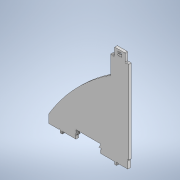
# Autodesk Inventor part: Support D - V2
Saved by Autodesk Inventor 2020 (Build 240168000, 168)
## iProperties
Created: 2020-07-22
Part Number: Support D - V2
Material: Generic
Document SubType Name: Modeling
Designer: Dan Wikman
Density: 1 g/cm^3
Appearance: Default
Author: Dan Wikman
Autodesk Inventor part; units mm, degrees
ref_plane "YZ Plane" through (0, 0, 0) normal (1, 0, 0) x (0, 1, 0)
ref_plane "XZ Plane" through (0, 0, 0) normal (0, 1, 0) x (-1, 0, 0)
ref_plane "XY Plane" through (0, 0, 0) normal (0, 0, 1) x (1, 0, 0)
sketch "Sketch1" plane through (0, 0, 0) normal (0, 0, 1) x (1, 0, 0)
  line L0 (-150, -512.3475) -> (-150, -323.3356) construction
  line L1 (-472.3938, -281.6809) -> (-252.3938, -281.6809) construction
  line L2 (-489.0365, 251.6809) -> (-252.3938, 251.6809) construction
  line L3 (-472.3938, 281.6809) -> (-252.3938, 281.6809) construction
  line L4 (-472.3938, -251.6809) -> (-252.3938, -251.6809) construction
  line L5 (-356.435, 15) -> (-576.435, 15) construction
  line L6 (-472.3938, -281.6809) -> (-472.3938, -251.6809) construction
  line L7 (-252.3938, -281.6809) -> (-252.3938, -251.6809) construction
  line L8 (-252.3938, 278.1809) -> (-252.3938, 251.6809) construction
  line L9 (-472.3938, 281.6809) -> (-472.3938, 251.6809) construction
  line L10 (-356.435, 15) -> (-356.435, -15) construction
  line L11 (-356.435, -15) -> (-576.435, -15) construction
  line L12 (-576.435, -15) -> (-576.435, 15) construction
  arc A0 (-150, -323.3356) -> (0, -356.435) centre (0, 0) ccw construction
  arc A1 (-156.5, -512.3475) -> (-160, -512.3475) centre (-158.25, -512.3475) ccw construction
  arc A2 (-190, -512.3475) -> (-193.5, -512.3475) centre (-191.75, -512.3475) ccw construction
  line L13 (-178.75, -519.0975) -> (-175, -519.0975) construction
  line L14 (-178.75, -529.0975) -> (-175, -529.0975) construction
  line L15 (-175, -519.0975) -> (-175, -529.0975) construction
  arc A3 (-178.75, -519.0975) -> (-178.75, -522.5975) centre (-178.75, -520.8475) ccw construction
  arc A4 (-178.75, -525.5975) -> (-178.75, -529.0975) centre (-178.75, -527.3475) ccw construction
  line L16 (-171.25, -519.0975) -> (-175, -519.0975) construction
  line L17 (-171.25, -529.0975) -> (-175, -529.0975) construction
  arc A5 (-171.25, -522.5975) -> (-171.25, -519.0975) centre (-171.25, -520.8475) ccw construction
  arc A6 (-171.25, -529.0975) -> (-171.25, -525.5975) centre (-171.25, -527.3475) ccw construction
  line L18 (-252.3938, 251.6809) -> (-489.0365, 251.6809) construction
  arc A7 (-334.9122, -265.623) -> (-335.582, -268.123) centre (-330.582, -268.123) ccw construction
  line L19 (-328.3782, -254.3059) -> (-334.9122, -265.623) construction
  arc A8 (-328.3782, -254.3059) -> (-329.8938, -251.6809) centre (-329.8938, -253.4309) ccw construction
  line L20 (-329.8938, -251.6809) -> (-394.8938, -251.6809) construction
  line L21 (-362.3938, -251.6809) -> (-362.3938, -293.6041) construction
  arc A9 (-389.2055, -268.123) -> (-389.8754, -265.623) centre (-394.2055, -268.123) ccw construction
  arc A10 (-394.8938, -251.6809) -> (-396.4093, -254.3059) centre (-394.8938, -253.4309) ccw construction
  line L22 (-396.4093, -254.3059) -> (-389.8754, -265.623) construction
  arc A11 (-389.2055, -291.6809) -> (-389.2055, -288.1809) centre (-389.2055, -289.9309) ccw construction
  line L23 (-389.2055, -291.6809) -> (-396.7055, -291.6809) construction
  line L24 (-396.7055, -281.6809) -> (-472.3938, -281.6809) construction
  line L25 (-328.082, -281.6809) -> (-252.3938, -281.6809) construction
  line L26 (-252.3938, -287.3475) -> (-210.8964, -287.3475) construction
  arc A12 (-210.8964, -287.3475) -> (-150, -323.3356) centre (0, 0) ccw construction
  arc A13 (-472.3938, -281.6809) -> (-246.475, -491.6809) centre (0, 0) ccw construction
  line L27 (-171.25, -436.0915) -> (-171.25, -399.5915) construction
  line L28 (-178.75, -436.0915) -> (-178.75, -399.5915) construction
  line L29 (-177, -437.8415) -> (-173, -437.8415) construction
  line L30 (-177, -397.8415) -> (-173, -397.8415) construction
  arc A14 (-177, -397.8415) -> (-178.75, -399.5915) centre (-177, -399.5915) ccw construction
  arc A15 (-178.75, -436.0915) -> (-177, -437.8415) centre (-177, -436.0915) ccw construction
  arc A16 (-173, -437.8415) -> (-171.25, -436.0915) centre (-173, -436.0915) ccw construction
  arc A17 (-171.25, -399.5915) -> (-173, -397.8415) centre (-173, -399.5915) ccw construction
  line L31 (-200, -512.3475) -> (-200, -491.6809) construction
  arc A18 (-200, -491.6809) -> (-203.5, -491.6809) centre (-201.75, -491.6809) ccw construction
  line L32 (-160, -512.3475) -> (-160, -532.5975) construction
  line L33 (-161.75, -534.3475) -> (-188.25, -534.3475) construction
  line L34 (-190, -532.5975) -> (-190, -512.3475) construction
  line L35 (-171.25, -522.5975) -> (-171.25, -525.5975) construction
  line L36 (-178.75, -522.5975) -> (-178.75, -525.5975) construction
  arc A19 (-190, -532.5975) -> (-188.25, -534.3475) centre (-188.25, -532.5975) ccw construction
  arc A20 (-161.75, -534.3475) -> (-160, -532.5975) centre (-161.75, -532.5975) ccw construction
  line L37 (-156.5, -512.3475) -> (-150, -512.3475) construction
  line L38 (-193.5, -512.3475) -> (-200, -512.3475) construction
  line L39 (-203.5, -491.6809) -> (-246.475, -491.6809) construction
  arc A21 (-396.7055, -288.1809) -> (-396.7055, -291.6809) centre (-396.7055, -289.9309) ccw construction
  line L40 (-396.7055, -281.6809) -> (-396.7055, -288.1809) construction
  line L41 (-389.2055, -288.1809) -> (-389.2055, -268.123) construction
  arc A22 (-335.582, -288.1809) -> (-335.582, -291.6809) centre (-335.582, -289.9309) ccw construction
  line L42 (-335.582, -291.6809) -> (-328.082, -291.6809) construction
  arc A23 (-328.082, -291.6809) -> (-328.082, -288.1809) centre (-328.082, -289.9309) ccw construction
  line L43 (-328.082, -281.6809) -> (-328.082, -288.1809) construction
  line L44 (-335.582, -288.1809) -> (-335.582, -268.123) construction
  arc A24 (-252.3938, -283.8475) -> (-252.3938, -287.3475) centre (-252.3938, -285.5975) ccw construction
  line L45 (-252.3938, -283.8475) -> (-252.3938, -281.6809) construction
  arc A25 (-479.7691, -25) -> (-479.7691, -21.5) centre (-479.7691, -23.25) ccw construction
  arc A26 (-479.7691, -1.4421) -> (-480.4389, 1.0579) centre (-484.7691, -1.4421) ccw construction
  line L46 (-486.9729, 12.375) -> (-480.4389, 1.0579) construction
  arc A27 (-485.4573, 15) -> (-486.9729, 12.375) centre (-485.4573, 13.25) ccw construction
  line L47 (-420.4573, 15) -> (-485.4573, 15) construction
  arc A28 (-425.4757, 1.0579) -> (-426.1456, -1.4421) centre (-421.1456, -1.4421) ccw construction
  arc A29 (-418.9418, 12.375) -> (-420.4573, 15) centre (-420.4573, 13.25) ccw construction
  line L48 (-418.9418, 12.375) -> (-425.4757, 1.0579) construction
  line L49 (-452.9573, 15) -> (-452.9573, -26.9232) construction
  line L50 (-479.7691, -25) -> (-487.2691, -25) construction
  line L51 (-487.2691, -15) -> (-549.7954, -15) construction
  arc A30 (-487.2691, -21.5) -> (-487.2691, -25) centre (-487.2691, -23.25) ccw construction
  line L52 (-487.2691, -15) -> (-487.2691, -21.5) construction
  line L53 (-479.7691, -21.5) -> (-479.7691, -1.4421) construction
  line L54 (-426.1456, -21.5) -> (-426.1456, -1.4421) construction
  arc A31 (-426.1456, -21.5) -> (-426.1456, -25) centre (-426.1456, -23.25) ccw construction
  line L55 (-426.1456, -25) -> (-418.6456, -25) construction
  arc A32 (-418.6456, -25) -> (-418.6456, -21.5) centre (-418.6456, -23.25) ccw construction
  line L56 (-418.6456, -15) -> (-418.6456, -21.5) construction
  line L57 (276.2049, -135.3556) -> (280.6774, -127.609)
  line L58 (279.2083, -124.984) -> (246.5502, -124.984)
  arc A33 (319.0505, -151.484) -> (319.0505, -147.984) centre (319.0505, -149.734) ccw
  arc A34 (328.5505, -147.9841) -> (325.0505, -147.9841) centre (326.8005, -147.9841) ccw
  line L59 (319.0505, -147.984) -> (280.8619, -147.984)
  arc A35 (214.0502, -164.7817) -> (212.5346, -167.4067) centre (214.0502, -166.5317) ccw
  arc A36 (280.5657, -167.4067) -> (279.0502, -164.7817) centre (279.0502, -166.5317) ccw
  arc A37 (274.0318, -178.7238) -> (273.3619, -181.2238) centre (278.3619, -181.2238) ccw
  line L60 (280.5657, -167.4067) -> (274.0318, -178.7238)
  line L61 (273.3619, -201.2817) -> (273.3619, -181.2238)
  arc A38 (273.3619, -201.2817) -> (273.3619, -204.7817) centre (273.3619, -203.0317) ccw
  line L62 (273.3619, -204.7817) -> (280.8619, -204.7817)
  arc A39 (280.8619, -204.7817) -> (280.8619, -201.2817) centre (280.8619, -203.0317) ccw
  line L63 (280.8619, -194.7817) -> (280.8619, -201.2817)
  line L64 (212.2384, -194.7817) -> (212.2384, -201.2817)
  arc A40 (212.2384, -201.2817) -> (212.2384, -204.7817) centre (212.2384, -203.0317) ccw
  arc A41 (219.7384, -204.7817) -> (219.7384, -201.2817) centre (219.7384, -203.0317) ccw
  line L65 (279.0502, -164.7817) -> (214.0502, -164.7817)
  line L66 (219.7384, -201.2817) -> (219.7384, -181.2238)
  line L67 (219.7384, -204.7817) -> (212.2384, -204.7817)
  arc A42 (219.7384, -181.2238) -> (219.0686, -178.7238) centre (214.7384, -181.2238) ccw
  line L68 (212.5346, -167.4067) -> (219.0686, -178.7238)
  line L69 (212.2384, -194.7817) -> (136.5502, -194.7817)
  line L70 (280.8619, -194.7817) -> (356.5502, -194.7817)
  line L71 (325.0505, -147.9841) -> (325.0505, -154.9841)
  line L72 (325.0505, -154.9841) -> (319.0505, -154.9841)
  line L73 (319.0505, -151.484) -> (319.0505, -154.9841)
  line L74 (246.5502, -124.984) -> (246.5502, -110.6064)
  arc A43 (280.6774, -127.609) -> (279.2083, -124.984) centre (279.1622, -126.7334) ccw
  arc A44 (280.8619, -138.8556) -> (280.8619, -135.3556) centre (280.8619, -137.1056) ccw
  line L75 (276.2049, -135.3556) -> (280.8619, -135.3556)
  line L76 (246.5502, -164.7817) -> (246.5502, -170.2759)
  line L77 (280.8619, -147.984) -> (280.8619, -138.8556)
  arc A45 (168.0499, -147.9841) -> (164.5499, -147.9841) centre (166.2999, -147.9841) ccw
  arc A46 (174.0499, -147.984) -> (174.0499, -151.484) centre (174.0499, -149.734) ccw
  line L78 (213.8921, -124.984) -> (246.5502, -124.984)
  line L79 (174.0499, -147.984) -> (212.2384, -147.984)
  line L80 (216.8955, -135.3556) -> (212.423, -127.609)
  line L81 (168.0499, -147.9841) -> (168.0499, -154.9841)
  line L82 (168.0499, -154.9841) -> (174.0499, -154.9841)
  line L83 (174.0499, -151.484) -> (174.0499, -154.9841)
  arc A47 (213.8921, -124.984) -> (212.423, -127.609) centre (213.9382, -126.7334) ccw
  arc A48 (212.2384, -135.3556) -> (212.2384, -138.8556) centre (212.2384, -137.1056) ccw
  line L84 (216.8955, -135.3556) -> (212.2384, -135.3556)
  line L85 (212.2384, -147.984) -> (212.2384, -138.8556)
  arc A49 (-280.3963, -274.7808) -> (-283.8935, -274.681) centre (-282.1435, -274.681) ccw construction
  arc A50 (-289.8935, -278.1809) -> (-289.8935, -274.6809) centre (-289.8935, -276.4309) ccw construction
  line L86 (-329.7357, -251.6809) -> (-362.3938, -251.6809) construction
  line L87 (-289.8935, -274.6809) -> (-328.082, -274.6809) construction
  line L88 (-332.7391, -262.0525) -> (-328.2666, -254.3059) construction
  line L89 (-283.8935, -274.681) -> (-283.8935, -281.681) construction
  line L90 (-283.8935, -281.681) -> (-289.8935, -281.681) construction
  line L91 (-289.8935, -278.1809) -> (-289.8935, -281.681) construction
  arc A51 (-328.2666, -254.3059) -> (-329.7357, -251.6809) centre (-329.7818, -253.4303) ccw construction
  arc A52 (-328.082, -265.5525) -> (-328.082, -262.0525) centre (-328.082, -263.8025) ccw construction
  line L92 (-332.7391, -262.0525) -> (-328.082, -262.0525) construction
  line L93 (-328.082, -274.6809) -> (-328.082, -265.5525) construction
  line L94 (-392.0485, -262.0525) -> (-396.7055, -262.0525) construction
  arc A53 (-396.7055, -262.0525) -> (-396.7055, -265.5525) centre (-396.7055, -263.8025) ccw construction
  line L95 (-392.0485, -262.0525) -> (-396.521, -254.3059) construction
  arc A54 (-395.0519, -251.6809) -> (-396.521, -254.3059) centre (-395.0058, -253.4303) ccw construction
  line L96 (-396.7055, -274.6809) -> (-396.7055, -265.5525) construction
  line L97 (-434.8941, -278.1809) -> (-434.8941, -281.681) construction
  line L98 (-434.8941, -274.6809) -> (-396.7055, -274.6809) construction
  arc A55 (-434.8941, -274.6809) -> (-434.8941, -278.1809) centre (-434.8941, -276.4309) ccw construction
  line L99 (-440.8941, -281.681) -> (-434.8941, -281.681) construction
  line L100 (-440.8941, -274.681) -> (-440.8941, -281.681) construction
  arc A56 (-440.8941, -274.681) -> (-444.3912, -274.7808) centre (-442.6441, -274.681) ccw construction
  line L101 (-395.0519, -251.6809) -> (-362.3938, -251.6809) construction
  line L102 (-444.3912, -274.7808) -> (-476.4404, -274.7808) construction
  arc A57 (-355.7859, -21.5) -> (-227.0273, -274.7808) centre (0, 0) ccw construction
  arc A58 (-549.7954, -15) -> (-476.4404, -274.7808) centre (0, 0) ccw construction
  line L103 (-280.3963, -274.7808) -> (-227.0273, -274.7808) construction
  line L104 (-364.1192, -15) -> (-364.1192, -18) construction
  arc A59 (-364.1192, -18) -> (-364.1192, -21.5) centre (-364.1192, -19.75) ccw construction
  line L105 (-364.1192, -21.5) -> (-355.7859, -21.5) construction
  line L106 (-356.1192, -15) -> (-356.435, -15) construction
  line L107 (-364.1192, -15) -> (-549.7954, -15) construction
  line L108 (-418.6456, -15) -> (-364.1192, -15) construction
  arc A60 (-370.957, -8.0002) -> (-374.457, -8.0002) centre (-372.707, -8.0002) ccw construction
  arc A61 (-380.457, -11.5) -> (-380.457, -8) centre (-380.457, -9.75) ccw construction
  line L109 (-420.2992, 15) -> (-452.9573, 15) construction
  line L110 (-380.457, -8) -> (-418.6456, -8) construction
  line L111 (-423.3026, 4.6284) -> (-418.8301, 12.375) construction
  line L112 (-374.457, -8.0002) -> (-374.457, -15.0002) construction
  line L113 (-374.457, -15.0002) -> (-380.457, -15.0002) construction
  line L114 (-380.457, -11.5) -> (-380.457, -15.0002) construction
  line L115 (-452.9573, 15) -> (-452.9573, 29.3776) construction
  arc A62 (-418.8301, 12.375) -> (-420.2992, 15) centre (-420.3453, 13.2506) ccw construction
  arc A63 (-418.6456, 1.1284) -> (-418.6456, 4.6284) centre (-418.6456, 2.8784) ccw construction
  line L116 (-423.3026, 4.6284) -> (-418.6456, 4.6284) construction
  line L117 (-418.6456, -8) -> (-418.6456, 1.1284) construction
  line L118 (-482.612, 4.6284) -> (-487.2691, 4.6284) construction
  arc A64 (-487.2691, 4.6284) -> (-487.2691, 1.1284) centre (-487.2691, 2.8784) ccw construction
  line L119 (-482.612, 4.6284) -> (-487.0845, 12.375) construction
  arc A65 (-485.6154, 15) -> (-487.0845, 12.375) centre (-485.5693, 13.2506) ccw construction
  line L120 (-487.2691, -8) -> (-487.2691, 1.1284) construction
  line L121 (-525.4576, -11.5) -> (-525.4576, -15.0002) construction
  line L122 (-525.4576, -8) -> (-487.2691, -8) construction
  arc A66 (-525.4576, -8) -> (-525.4576, -11.5) centre (-525.4576, -9.75) ccw construction
  line L123 (-531.4576, -15.0002) -> (-525.4576, -15.0002) construction
  line L124 (-531.4576, -8.0002) -> (-531.4576, -15.0002) construction
  arc A67 (-531.4576, -8.0002) -> (-534.9576, -8.0002) centre (-533.2076, -8.0002) ccw construction
  line L125 (-485.6154, 15) -> (-452.9573, 15) construction
  line L126 (-370.957, -8.0002) -> (-356.3452, -8.0002) construction
  line L127 (-534.9576, -8.0002) -> (-549.9418, -8.0002) construction
  line L128 (-328.082, 251.6809) -> (-328.082, 245.1809) construction
  arc A68 (-328.082, 241.6809) -> (-328.082, 245.1809) centre (-328.082, 243.4309) ccw construction
  line L129 (-396.7055, 251.6809) -> (-396.7055, 245.1809) construction
  arc A69 (-396.7055, 245.1809) -> (-396.7055, 241.6809) centre (-396.7055, 243.4309) ccw construction
  arc A70 (-389.2055, 241.6809) -> (-389.2055, 245.1809) centre (-389.2055, 243.4309) ccw construction
  line L130 (-389.2055, 245.1809) -> (-389.2055, 265.2388) construction
  line L131 (-389.2055, 241.6809) -> (-396.7055, 241.6809) construction
  arc A71 (-389.2055, 265.2388) -> (-389.8754, 267.7388) centre (-394.2055, 265.2388) ccw construction
  line L132 (-396.4093, 279.0559) -> (-389.8754, 267.7388) construction
  arc A72 (-394.8938, 281.6809) -> (-396.4093, 279.0559) centre (-394.8938, 279.9309) ccw construction
  line L133 (-329.8938, 281.6809) -> (-394.8938, 281.6809) construction
  arc A73 (-334.9122, 267.7388) -> (-335.582, 265.2388) centre (-330.582, 265.2388) ccw construction
  arc A74 (-328.3782, 279.0559) -> (-329.8938, 281.6809) centre (-329.8938, 279.9309) ccw construction
  line L134 (-328.3782, 279.0559) -> (-334.9122, 267.7388) construction
  arc A75 (-335.582, 245.1809) -> (-335.582, 241.6809) centre (-335.582, 243.4309) ccw construction
  line L135 (-335.582, 241.6809) -> (-328.082, 241.6809) construction
  line L136 (-335.582, 245.1809) -> (-335.582, 265.2388) construction
  line L137 (-328.082, 251.6809) -> (-252.3938, 251.6809) construction
  line L138 (-396.7055, 251.6809) -> (-472.3938, 251.6809) construction
  line L139 (-362.3938, 281.6809) -> (-362.3938, 276.1867) construction
  line L140 (-472.3938, 251.6809) -> (-472.3938, 248.6809) construction
  arc A76 (-472.3938, 245.1809) -> (-472.3938, 248.6809) centre (-472.3938, 246.9309) ccw construction
  line L141 (-472.3938, 245.1809) -> (-492.3275, 245.1809) construction
  arc A77 (-492.3275, 245.1809) -> (-549.7954, 15) centre (0, 0) ccw construction
  arc A78 (-252.3938, 251.6809) -> (-356.3452, -8.0002) centre (0, 0) ccw construction
  line L142 (-549.7954, 15) -> (-576.435, 15) construction
  line L143 (-576.435, 15) -> (-576.435, -8.0002) construction
  line L144 (-549.9418, -8.0002) -> (-576.435, -8.0002) construction
  arc A79 (-280.3935, 258.6807) -> (-283.8935, 258.6807) centre (-282.1435, 258.6807) ccw
  arc A80 (-289.8935, 255.1809) -> (-289.8935, 258.6809) centre (-289.8935, 256.9309) ccw
  line L145 (-329.7357, 281.6809) -> (-362.3823, 281.6809)
  line L146 (-289.8935, 258.6809) -> (-328.082, 258.6809)
  line L147 (-332.7391, 271.3093) -> (-328.2666, 279.0559)
  line L148 (-283.8935, 258.6807) -> (-283.8935, 251.6807)
  line L149 (-283.8935, 251.6807) -> (-289.8935, 251.6807)
  line L150 (-289.8935, 255.1809) -> (-289.8935, 251.6807)
  line L151 (-362.3823, 281.6809) -> (-362.3823, 296.0585)
  arc A81 (-328.2666, 279.0559) -> (-329.7357, 281.6809) centre (-329.7818, 279.9315) ccw
  arc A82 (-328.082, 267.8093) -> (-328.082, 271.3093) centre (-328.082, 269.5593) ccw
  line L152 (-332.7391, 271.3093) -> (-328.082, 271.3093)
  line L153 (-328.082, 258.6809) -> (-328.082, 267.8093)
  line L154 (-392.0255, 271.3093) -> (-396.6826, 271.3093)
  arc A83 (-396.6826, 271.3093) -> (-396.6826, 267.8093) centre (-396.6826, 269.5593) ccw
  line L155 (-392.0255, 271.3093) -> (-396.498, 279.0559)
  arc A84 (-395.0289, 281.6809) -> (-396.498, 279.0559) centre (-394.9828, 279.9315) ccw
  line L156 (-396.6826, 258.6809) -> (-396.6826, 267.8093)
  line L157 (-434.8711, 255.1809) -> (-434.8711, 251.6807)
  line L158 (-434.8711, 258.6809) -> (-396.6826, 258.6809)
  arc A85 (-434.8711, 258.6809) -> (-434.8711, 255.1809) centre (-434.8711, 256.9309) ccw
  line L159 (-440.8711, 251.6807) -> (-434.8711, 251.6807)
  line L160 (-440.8711, 258.6807) -> (-440.8711, 251.6807)
  arc A86 (-440.8711, 258.6807) -> (-444.3711, 258.6807) centre (-442.6211, 258.6807) ccw
  line L161 (-395.0289, 281.6809) -> (-362.3823, 281.6809)
  line L162 (-444.3711, 258.6807) -> (-472.3938, 258.6807)
  line L163 (-280.3935, 258.6807) -> (-252.3938, 258.6807)
  line L164 (-252.3938, 258.6807) -> (-252.3938, 278.1809)
  line L165 (-252.3938, 281.6809) -> (-218.4073, 281.6809)
  arc A87 (-252.3938, 281.6809) -> (-252.3938, 278.1809) centre (-252.3938, 279.9309) ccw
  arc A88 (-271.25, 519.0975) -> (-271.25, 522.5975) centre (-271.25, 520.8475) ccw
  line L166 (-271.25, 519.0975) -> (-275, 519.0975)
  arc A89 (-271.25, 525.5975) -> (-271.25, 529.0975) centre (-271.25, 527.3475) ccw
  line L167 (-278.75, 519.0975) -> (-275, 519.0975)
  line L168 (-271.25, 529.0975) -> (-275, 529.0975)
  line L169 (-275, 519.0975) -> (-275, 529.0975)
  line L170 (-278.75, 529.0975) -> (-275, 529.0975)
  line L171 (-275, 534.3475) -> (-275, 537.9358)
  line L172 (-261.3333, 534.3475) -> (-288.6667, 534.3475)
  arc A90 (-260, 512.3475) -> (-256.5, 512.3475) centre (-258.25, 512.3475) ccw
  arc A91 (-293.5, 512.3475) -> (-290, 512.3475) centre (-291.75, 512.3475) ccw
  arc A92 (-278.75, 522.5975) -> (-278.75, 519.0975) centre (-278.75, 520.8475) ccw
  arc A93 (-278.75, 529.0975) -> (-278.75, 525.5975) centre (-278.75, 527.3475) ccw
  arc A94 (-288.6667, 534.3475) -> (-290, 533.0142) centre (-288.2908, 532.6384) ccw
  arc A95 (-260, 533.0142) -> (-261.3333, 534.3475) centre (-261.7092, 532.6384) ccw
  arc A96 (-291.7627, 515.4872) -> (-291.9051, 515.4342) centre (-100, 0) ccw
  line L173 (-250, 512.3475) -> (-250, 281.6809)
  line L174 (-300, 512.3475) -> (-300, 460.9772)
  arc A97 (-300, 460.9772) -> (-472.3938, 281.6809) centre (0, 0) ccw
  line L175 (-219.7787, 527.0975) -> (-219.7787, 529.0975)
  line L176 (-250, 512.3475) -> (-256.5, 512.3475)
  line L177 (-293.5, 512.3475) -> (-300, 512.3475)
  line L178 (-260, 533.0142) -> (-260, 512.3475)
  line L179 (-290, 533.0142) -> (-290, 512.3475)
  line L180 (-278.75, 522.5975) -> (-278.75, 525.5975)
  line L181 (-271.25, 525.5975) -> (-271.25, 522.5975)
  line L182 (-472.3938, 258.6807) -> (-472.3938, 281.6809)
  arc A98 (-485.3702, 258.6809) -> (-485.3703, 258.6807) centre (0, 0) ccw
  line L183 (-247.8856, -513.2316) -> (-248.7643, -288.2333) projected
  line L184 (-251.1802, -282.576) -> (-326.8679, -282.8716) projected
  point P0 (0, -512.3475)
  point P1 (-190, -534.3475)
  point P2 (-160, -534.3475)
  point P3 (-59.9119, -534.1417)
  point P4 (-389.2055, -259.0142)
  point P5 (-479.7691, 7.6667)
  point P6 (328.5476, -148.0839)
  point P7 (328.0311, -152.0673)
  point P8 (329.3645, -149.3173)
  point P9 (219.7384, -172.1151)
  point P10 (164.5527, -148.0839)
  point P11 (165.0692, -152.0673)
  point P12 (163.7359, -149.3173)
  point P13 (-280.9128, -278.7642)
  point P14 (-279.5795, -276.0142)
  point P15 (-443.8747, -278.7642)
  point P16 (-445.2081, -276.0142)
  point P17 (-370.9599, -8.1)
  point P18 (-371.4764, -12.0833)
  point P19 (-370.143, -9.3333)
  point P20 (-534.4382, -12.0833)
  point P21 (-534.9548, -8.1)
  point P22 (-535.7716, -9.3333)
  point P23 (-389.2055, 274.3475)
  point P24 (-280.3733, 258.5809)
  point P25 (-280.8899, 254.5975)
  point P26 (-279.5565, 257.3475)
  point P27 (-443.8747, 254.5975)
  point P28 (-444.3912, 258.5809)
  point P29 (-445.2081, 257.3475)
  point P30 (-290, 534.3475)
  point P31 (-260, 534.3475)
  dimension "d19" = 150
  dimension "d54" = 220
  dimension "d56" = 220
  dimension "d57" = 30
  dimension "d59" = 30
  dimension "d73" = 236.6809
  dimension "d74" = 236.6809
  dimension "d75" = 576.435
  dimension "d76" = 472.3938
  dimension "d77" = 472.3938
  dimension "d78" = 30
  dimension "d82" = 252.3938
  dimension "d85" = 356.435
  dimension "d88" = 3.5
  dimension "d89" = 30
  dimension "d90" = 22
  dimension "d91" = 3.5
  dimension "d103" = 3.75
  dimension "d104" = 3.75
  dimension "d134" = 3.5
  dimension "d135" = 65
  dimension "d136" = 65
  dimension "d137" = 7.3333
  dimension "d138" = 60
  dimension "d139" = 5
  dimension "d140" = 7.5
  dimension "d148" = 1.75
  dimension "d151" = 40
  dimension "d152" = 74.506
  dimension "d153" = 20.6667
  dimension "d154" = 3.5
  dimension "d155" = 189.012
  dimension "d159" = 1.75
  dimension "d160" = 1.75
  dimension "d161" = 1.75
  dimension "d164" = 7.5
  dimension "d168" = 21.25
  dimension "d170" = 30
  dimension "d171" = 1.75
  dimension "d172" = 10
  dimension "d173" = 3.5
  dimension "d177" = 3.5
  dimension "d178" = 65
  dimension "d179" = 65
  dimension "d180" = 7.3333
  dimension "d181" = 60
  dimension "d182" = 5
  dimension "d183" = 7.5
  dimension "d185" = 1.75
  dimension "d186" = 10
  dimension "d192" = 1.75
  dimension "d206" = 1.75
  dimension "d208" = 220
  dimension "d209" = 3.5
  dimension "d210" = 65
  dimension "d211" = 65
  dimension "d212" = 7.3333
  dimension "d213" = 60
  dimension "d214" = 5
  dimension "d215" = 7.5
  dimension "d216" = 30
  dimension "d217" = 1.75
  dimension "d218" = 10
  dimension "d219" = 7
  constraints: 366 end point, 203 point on circle, 99 centre point, 90 symmetric about line, 40 vertical, 33 tangent, 27 horizontal, 17 perpendicular, 15 point on line, 5 midpoint, 4 collinear, 4 equal radius, 4 parallel, 2 coincident, 36 other
  measures "d19" distance from line of point (0, 0) L0
  measures "d54" distance of L5.start L5.end
  measures "d56" distance of L1.start L1.end
  measures "d57" distance of L1.end L4.end
  measures "d59" distance between parallel lines of L3 L2
  measures "d73" distance between parallel lines of L4 L11
  measures "d74" distance between parallel lines of L2 L5
  measures "d75" distance from line of L12 point (0, 0)
  measures "d76" distance from line of point (0, 0) L6
  measures "d77" distance from line of point (0, 0) L9
  measures "d78" distance of L5.start L10.end
  measures "d82" distance from line of point (0, 0) L8
  measures "d85" distance from line of A13.centre L10
  measures "d88" diameter of A1
  measures "d89" distance of point (-190, -534.348) point (-160, -534.348)
  measures "d90" distance of point (-160, -534.348) L32.start
  measures "d91" diameter of A2
  measures "d103" distance of L13.start L13.end
  measures "d104" distance of L14.start L14.end
  measures "d134" diameter of A8
  measures "d135" distance of L20.start L20.end
  measures "d136" distance between centres of A8 A10
  measures "d137" distance from line of point (-389.206, -259.014) L20
  measures "d138" angle of L20 L22
  measures "d139" radius of A9
  measures "d140" distance of L23.start L23.end
  measures "d148" radius of A14
  measures "d151" distance between parallel lines of L29 L30
  measures "d152" distance from line of L0.end L30
  measures "d153" distance of L31.start L31.end
  measures "d154" diameter of A18
  measures "d155" distance of L0.start L0.end
  measures "d159" radius of A3
  measures "d160" radius of A6
  measures "d161" radius of A19
  measures "d164" distance between parallel lines of L28 L27
  measures "d168" distance between parallel lines of L27 L0
  measures "d170" distance between parallel lines of L25 L20
  measures "d171" radius of A11
  measures "d172" distance between parallel lines of L24 L23
  measures "d173" diameter of A24
  measures "d177" diameter of A29
  measures "d178" distance of L47.start L47.end
  measures "d179" distance between centres of A29 A27
  measures "d180" distance from line of point (-479.769, 7.667) L47
  measures "d181" angle of L47 L46
  measures "d182" radius of A26
  measures "d183" distance of L50.start L50.end
  measures "d185" radius of A25
  measures "d186" distance between parallel lines of L51 L50
  measures "d192" radius of A33
  measures "d206" radius of A34
  measures "d208" distance of L69.end L70.end
  measures "d209" diameter of A36
  measures "d210" distance of L65.start L65.end
  measures "d211" distance between centres of A36 A35
  measures "d212" distance from line of point (219.738, -172.115) L65
  measures "d213" angle of L65 L68
  measures "d214" radius of A42
  measures "d215" distance of L67.start L67.end
  measures "d216" distance between parallel lines of L70 L65
  measures "d217" radius of A41
  measures "d218" distance between parallel lines of L69 L67
  measures "d219" distance of L71.start L71.end
extrude "Extrusion4" add sketch "Sketch1" along normal blind 7 contours A79 L148 L149 L150 A80 L146 L153 A82 L152 L147 A81 L145 L161 A84 L155 L154 A83 L156 L158 A85 L157 L159 L160 A86 L162 L182 A97 A98 L173 L165 A87 L164 L163 | A98 L174 L177 A91 L179 A94 L172 A95 L178 A90 L176 L173
body "Solid4"
